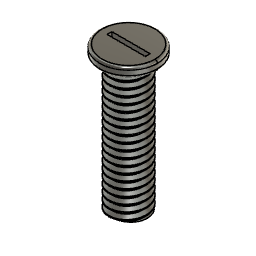
Modelo_Tornillo (Autodesk Fusion 360 design; units mm, degrees)
Autodesk Fusion 360 part; units mm, degrees
cylinder "CilindroPrimitivo1" add diameter 4.5 height 14 placed x (1, 0, 0) y (0, 1, 0) z (0, 0, 1) at (0, 0, 0) makes body 1
sketch "Boceto2" plane through (0, 0, 14) normal (0, 0, 1) x (-1, 0, 0)
  circle A0 centre (0, 0) radius 2.25
  circle A1 centre (0, 0) radius 3
  dimension "d5" = 6
  constraint coincident A0.centre A1.centre
  measures "d5" diameter of A1
extrude "Extruir1" add sketch "Boceto2" along normal blind 1 separate body contours A0 | A1 makes body 2
thread "Rosca1" "ISO Metric profile 4.0 M4x0.7 6g" major diameter 3.908 minor diameter 3.111 pitch 0.7 angle 60 modelled right hand crest width 0.1017 on face at (2.2388, -0.224, 4.6667) crest through (1.954, 0, -0.175) on bodies 1
fillet "Empalme1" radius 0.25 curvature continuous 2 edges at (2.797, 1.0848, 15) (2.797, 1.0848, 14) on bodies 2
sketch "Boceto3" plane through (0, 0, 15) normal (0, 0, 1) x (-1, 0, 0)
  circle A0 centre (0, 0) radius 2.75
  line L0 (2.75, 0) -> (-2.75, 0) construction
  line L1 (0, -3) -> (0, 3) construction
  line L2 (2, 0.25) -> (-2, 0.25)
  line L3 (-2, 0.25) -> (-2, -0.25)
  line L4 (-2, -0.25) -> (2, -0.25)
  line L5 (2, -0.25) -> (2, 0.25)
  line L6 (2, 0.25) -> (-2, -0.25) construction
  line L7 (-2, 0.25) -> (2, -0.25) construction
  dimension "d10" = 4
  dimension "d11" = 0.5
  constraint coincident A0 L0.start
  constraint coincident A0 L0.end
  constraint horizontal L0
  constraint perpendicular L0 L1
  constraint horizontal L2
  constraint perpendicular L2 L3
  constraint parallel L2 L4
  constraint parallel L3 L5
  constraint coincident L6 A0.centre
  constraint coincident L7 A0.centre
  constraint coincident A0.centre origin
  measures "d10" distance of L3.end L4.end
  measures "d11" distance of L2.end L3.end
extrude "Extruir2" cut sketch "Boceto3" against normal blind 0.5 contours L2 L3 L4 L5 bodies 2
combine "Combinar1" operation add target body 1 tool bodies 2
